Autodesk Fusion 360 part; units mm, degrees
(part 7 of 7)
  measures "d140" distance of A39.centre L1475
  measures "d141" diameter of A36
  measures "d142" distance of A36.centre L3866
  measures "d143" distance of A36.centre L1475
  measures "d144" diameter of A2
  measures "d145" distance of A0.centre L214
  measures "d146" distance of A0.centre L904
  measures "d147" diameter of A29
  measures "d148" distance of A21.centre L241
  measures "d149" distance of A21.centre L1147
  measures "d150" diameter of A17
  measures "d151" distance of A17.centre L2172
  measures "d152" distance of A17.centre L1106
  measures "d153" diameter of A69
  measures "d154" diameter of A50
  measures "d155" diameter of A63
  measures "d156" diameter of A15
  measures "d157" diameter of A47
  measures "d158" diameter of A5
  measures "d159" distance of A5.centre L1493
  measures "d160" distance of A43.centre L926
  measures "d161" distance of A15.centre L926
  measures "d162" distance of A60.centre L796
  measures "d163" distance of A68.centre L4112
  measures "d164" distance of A17.centre L1102
  measures "d165" distance of A68.centre L4388
  measures "d166" distance of A68.centre L4363
  measures "d167" distance of A49.centre L3076
  measures "d168" distance of A49.centre L3488
  measures "d169" distance of A60.centre L3636
  measures "d170" distance of A60.centre L3768
  measures "d171" distance of A15.centre L1414
  measures "d172" distance of A15.centre L1372
  measures "d173" distance of A43.centre L577
  measures "d174" distance of A43.centre L2522
  measures "d175" distance of A5.centre L729
  measures "d176" distance of A5.centre L761
  measures "d177" distance of A17.centre L1070
  measures "d178" distance of A17.centre L1079
  measures "d179" distance of A21.centre L1134
  measures "d180" distance of A21.centre L1105
  measures "d181" distance of A0.centre L205
  measures "d182" distance of A0.centre L871
  measures "d183" distance of A53.centre L2428
  measures "d184" distance of A53.centre L3199
  measures "d185" distance of A39.centre L4631
  measures "d186" distance of A39.centre L1477
  measures "d187" distance of A36.centre L1441
  measures "d188" radius of A32
  measures "d189" distance of L2406 L2562
  measures "d190" distance of L2398 L2487
  measures "d191" distance of L2399 L2562
  measures "d192" distance of L2398 L2532
  measures "d193" distance of L2406 L2546
  measures "d194" distance of L2487 L2580
  measures "d195" distance of L2490 L2532
  measures "d196" distance of L1493 L2399
sketch "Sketch3" plane through (0, 0, 0) normal (0, 0, 1) x (1, 0, 0)
  line L0 (-169.0689, -23.2426) -> (259.656, -23.2426)
  arc A0 (-174.0689, -18.2426) -> (-169.0689, -23.2426) centre (-169.0689, -18.2426) ccw
  line L1 (-174.0689, 118.4832) -> (-174.0689, -18.2426)
  arc A1 (-169.0689, 123.4832) -> (-174.0689, 118.4832) centre (-169.0689, 118.4832) ccw
  line L2 (-158.7961, 123.4832) -> (-169.0689, 123.4832)
  line L3 (259.656, 123.4832) -> (-158.7961, 123.4832)
  arc A2 (264.656, 118.4832) -> (259.656, 123.4832) centre (259.656, 118.4832) ccw
  line L4 (264.656, -18.2426) -> (264.656, 118.4832)
  arc A3 (259.656, -23.2426) -> (264.656, -18.2426) centre (259.656, -18.2426) ccw
  line L5 (260.257, 83.109) -> (260.257, -11.1417)
  line L6 (257.232, 0.4083) -> (257.232, 14.4091)
  line L7 (209.607, -9.1167) -> (195.605, -9.1167)
  line L8 (162.267, 109.6602) -> (176.267, 109.6602)
  line L9 (-166.345, 99.7592) -> (-166.345, 105.5592)
  line L10 (205.13, 81.084) -> (219.132, 81.084)
  line L11 (143.217, 95.6582) -> (157.217, 95.6582)
  line L12 (121.142, 83.109) -> (121.142, -11.1417)
  line L13 (114.998, -11.1417) -> (114.998, 83.109)
  line L14 (183.055, 83.109) -> (183.055, -11.1417)
  line L15 (179.292, -11.1417) -> (179.292, 83.109)
  line L16 (-131.2701, 111.6852) -> (-131.2701, 93.6332)
  line L17 (-149.3191, 93.6332) -> (-149.3191, 111.6852)
  line L18 (-45.545, 111.6852) -> (-45.545, 93.6332)
  line L19 (-54.069, 93.6332) -> (-54.069, 111.6852)
  line L20 (40.18, 111.6852) -> (40.18, 93.6332)
  line L21 (31.656, 93.6332) -> (31.656, 111.6852)
  line L22 (121.142, 111.6852) -> (121.142, 93.6332)
  line L23 (117.381, 93.6332) -> (117.381, 111.6852)
  line L24 (179.292, 93.6332) -> (179.292, 111.6852)
  line L25 (185.808, 109.3822) -> (198.508, 109.3822)
  line L26 (185.808, 96.3822) -> (185.808, 109.3822)
  line L27 (198.508, 96.3822) -> (185.808, 96.3822)
  line L28 (198.508, 109.3822) -> (198.508, 96.3822)
  line L29 (-152.3441, 99.7592) -> (-152.3441, 105.5592)
  line L30 (-128.2451, 105.5592) -> (-128.2451, 99.7592)
  line L31 (43.205, 99.7592) -> (43.205, 105.5592)
  line L32 (114.356, 105.5592) -> (114.356, 99.7592)
  line L33 (-57.094, 99.7592) -> (-57.094, 105.5592)
  line L34 (-42.52, 99.7592) -> (-42.52, 105.5592)
  line L35 (28.631, 105.5592) -> (28.631, 99.7592)
  line L36 (124.167, 105.5592) -> (124.167, 99.7592)
  line L37 (176.267, 105.5592) -> (176.267, 99.7592)
  line L38 (186.08, 52.1344) -> (186.08, 57.9344)
  line L39 (176.267, 57.9344) -> (176.267, 52.1344)
  line L40 (111.973, -5.0157) -> (111.973, 0.7845)
  line L41 (124.167, -5.0157) -> (124.167, 0.7845)
  line L42 (-168.37, 112.6852) -> (-150.3191, 112.6852)
  line L43 (-168.37, 92.6332) -> (-150.3191, 92.6332)
  line L44 (-130.2701, 92.6332) -> (-55.069, 92.6332)
  line L45 (-130.2701, 112.6852) -> (-55.069, 112.6852)
  line L46 (-44.545, 92.6332) -> (30.656, 92.6332)
  line L47 (-44.545, 112.6852) -> (30.656, 112.6852)
  line L48 (41.18, 92.6332) -> (116.381, 92.6332)
  line L49 (122.142, 92.6332) -> (178.292, 92.6332)
  line L50 (113.998, 84.109) -> (-168.37, 84.109)
  line L51 (41.18, 112.6852) -> (116.381, 112.6852)
  line L52 (122.142, 112.6852) -> (178.292, 112.6852)
  line L53 (259.257, 84.109) -> (184.055, 84.109)
  line L54 (178.292, 84.109) -> (122.142, 84.109)
  line L55 (259.257, -12.1417) -> (184.055, -12.1417)
  line L56 (178.292, -12.1417) -> (122.142, -12.1417)
  line L57 (113.998, -12.1417) -> (-168.37, -12.1417)
  line L58 (-169.37, -11.1417) -> (-169.37, 83.109)
  line L59 (-169.37, 93.6332) -> (-169.37, 111.6852)
  line L60 (185.808, 109.3822) -> (198.508, 96.3822)
  circle A4 centre (192.158, 102.8822) radius 3.75
  circle A5 centre (192.158, 102.8822) radius 9.25
  arc A6 (-168.37, 112.6852) -> (-169.37, 111.6852) centre (-168.37, 111.6852) ccw
  arc A7 (-169.37, 93.6332) -> (-168.37, 92.6332) centre (-168.37, 93.6332) ccw
  arc A8 (-150.3191, 92.6332) -> (-149.3191, 93.6332) centre (-150.3191, 93.6332) ccw
  arc A9 (-149.3191, 111.6852) -> (-150.3191, 112.6852) centre (-150.3191, 111.6852) ccw
  arc A10 (-130.2701, 112.6852) -> (-131.2701, 111.6852) centre (-130.2701, 111.6852) ccw
  arc A11 (-131.2701, 93.6332) -> (-130.2701, 92.6332) centre (-130.2701, 93.6332) ccw
  arc A12 (-54.069, 111.6852) -> (-55.069, 112.6852) centre (-55.069, 111.6852) ccw
  arc A13 (-55.069, 92.6332) -> (-54.069, 93.6332) centre (-55.069, 93.6332) ccw
  arc A14 (-45.545, 93.6332) -> (-44.545, 92.6332) centre (-44.545, 93.6332) ccw
  arc A15 (-44.545, 112.6852) -> (-45.545, 111.6852) centre (-44.545, 111.6852) ccw
  arc A16 (31.656, 111.6852) -> (30.656, 112.6852) centre (30.656, 111.6852) ccw
  arc A17 (30.656, 92.6332) -> (31.656, 93.6332) centre (30.656, 93.6332) ccw
  arc A18 (40.18, 93.6332) -> (41.18, 92.6332) centre (41.18, 93.6332) ccw
  arc A19 (41.18, 112.6852) -> (40.18, 111.6852) centre (41.18, 111.6852) ccw
  arc A20 (117.381, 111.6852) -> (116.381, 112.6852) centre (116.381, 111.6852) ccw
  arc A21 (116.381, 92.6332) -> (117.381, 93.6332) centre (116.381, 93.6332) ccw
  arc A22 (121.142, 93.6332) -> (122.142, 92.6332) centre (122.142, 93.6332) ccw
  arc A23 (122.142, 112.6852) -> (121.142, 111.6852) centre (122.142, 111.6852) ccw
  arc A24 (179.292, 111.6852) -> (178.292, 112.6852) centre (178.292, 111.6852) ccw
  arc A25 (178.292, 92.6332) -> (179.292, 93.6332) centre (178.292, 93.6332) ccw
  arc A26 (184.055, 84.109) -> (183.055, 83.109) centre (184.055, 83.109) ccw
  arc A27 (260.257, 83.109) -> (259.257, 84.109) centre (259.257, 83.109) ccw
  arc A28 (259.257, -12.1417) -> (260.257, -11.1417) centre (259.257, -11.1417) ccw
  arc A29 (183.055, -11.1417) -> (184.055, -12.1417) centre (184.055, -11.1417) ccw
  arc A30 (179.292, 83.109) -> (178.292, 84.109) centre (178.292, 83.109) ccw
  arc A31 (178.292, -12.1417) -> (179.292, -11.1417) centre (178.292, -11.1417) ccw
  arc A32 (121.142, -11.1417) -> (122.142, -12.1417) centre (122.142, -11.1417) ccw
  arc A33 (122.142, 84.109) -> (121.142, 83.109) centre (122.142, 83.109) ccw
  arc A34 (114.998, 83.109) -> (113.998, 84.109) centre (113.998, 83.109) ccw
  arc A35 (113.998, -12.1417) -> (114.998, -11.1417) centre (113.998, -11.1417) ccw
  arc A36 (-169.37, -11.1417) -> (-168.37, -12.1417) centre (-168.37, -11.1417) ccw
  arc A37 (-168.37, 84.109) -> (-169.37, 83.109) centre (-168.37, 83.109) ccw
  line L61 (-152.3441, 109.6602) -> (-166.345, 109.6602)
  line L62 (-166.345, 95.6582) -> (-152.3441, 95.6582)
  line L63 (-171.5689, 114.6832) -> (262.156, 114.6832)
  line L64 (-171.5689, 114.6832) -> (-171.5689, -14.4426)
  line L65 (262.156, -14.4426) -> (-171.5689, -14.4426)
  line L66 (262.156, 114.6832) -> (262.156, -14.4426)
  dimension "d197" = 3.025
  dimension "d198" = 3.025
  dimension "d199" = 3.025
  dimension "d200" = 3.025
  dimension "d201" = 3.025
  dimension "d202" = 3.025
  dimension "d203" = 3.025
  dimension "d204" = 3.025
  dimension "d205" = 3.025
  dimension "d206" = 3.025
  dimension "d207" = 3.025
  dimension "d208" = 3.025
  dimension "d209" = 3.025
  dimension "d210" = 3.025
  dimension "d211" = 3.025
  dimension "d212" = 3.025
  dimension "d213" = 3.025
  dimension "d214" = 3.025
  dimension "d215" = 3.025
  dimension "d216" = 7.5
  dimension "d218" = 18.5
  dimension "d219" = 1
  constraint horizontal L42
  constraint vertical L5
  constraint horizontal L55
  constraint vertical L58
  constraint horizontal L43
  constraint horizontal L53
  constraint vertical L12
  constraint vertical L13
  constraint vertical L14
  constraint vertical L15
  constraint vertical L16
  constraint vertical L17
  constraint vertical L18
  constraint vertical L19
  constraint vertical L20
  constraint vertical L21
  constraint vertical L22
  constraint vertical L23
  constraint vertical L24
  constraint collinear L42 L45
  constraint collinear L43 L44
  constraint collinear L44 L46
  constraint collinear L45 L47
  constraint collinear L46 L48
  constraint collinear L47 L51
  constraint collinear L48 L49
  constraint collinear L50 L54
  constraint collinear L51 L52
  constraint collinear L53 L54
  constraint collinear L55 L56
  constraint collinear L56 L57
  constraint collinear L58 L59
  constraint coincident L25.start L26.end
  constraint coincident L27.start L28.end
  constraint midpoint L60 A4.centre
  constraint tangent L42 A6
  constraint tangent L59 A6
  constraint tangent L43 A7
  constraint tangent L59 A7
  constraint equal A6 A7
  constraint tangent L17 A8
  constraint tangent L43 A8
  constraint equal A6 A8
  constraint tangent L17 A9
  constraint tangent L42 A9
  constraint equal A6 A9
  constraint tangent L16 A10
  constraint tangent L45 A10
  constraint equal A6 A10
  constraint tangent L16 A11
  constraint tangent L44 A11
  constraint equal A6 A11
  constraint tangent L19 A12
  constraint tangent L45 A12
  constraint equal A6 A12
  constraint tangent L19 A13
  constraint tangent L44 A13
  constraint equal A6 A13
  constraint tangent L18 A14
  constraint tangent L46 A14
  constraint equal A6 A14
  constraint tangent L18 A15
  constraint tangent L47 A15
  constraint equal A6 A15
  constraint tangent L21 A16
  constraint tangent L47 A16
  constraint equal A6 A16
  constraint tangent L21 A17
  constraint tangent L46 A17
  constraint equal A6 A17
  constraint tangent L20 A18
  constraint tangent L48 A18
  constraint equal A6 A18
  constraint tangent L20 A19
  constraint tangent L51 A19
  constraint equal A6 A19
  constraint tangent L23 A20
  constraint tangent L51 A20
  constraint equal A6 A20
  constraint tangent L23 A21
  constraint tangent L48 A21
  constraint equal A6 A21
  constraint tangent L22 A22
  constraint tangent L49 A22
  constraint equal A6 A22
  constraint tangent L22 A23
  constraint tangent L52 A23
  constraint equal A6 A23
  constraint tangent L52 A24
  constraint tangent L24 A24
  constraint equal A6 A24
  constraint tangent L49 A25
  constraint tangent L24 A25
  constraint equal A6 A25
  constraint tangent L53 A26
  constraint tangent L14 A26
  constraint equal A6 A26
  constraint tangent L53 A27
  constraint tangent L5 A27
  constraint equal A6 A27
  constraint tangent L5 A28
  constraint tangent L55 A28
  constraint equal A6 A28
  constraint tangent L55 A29
  constraint tangent L14 A29
  constraint equal A6 A29
  constraint tangent L15 A30
  constraint tangent L54 A30
  constraint equal A6 A30
  constraint tangent L15 A31
  constraint tangent L56 A31
  constraint equal A6 A31
  constraint tangent L56 A32
  constraint tangent L12 A32
  constraint equal A6 A32
  constraint tangent L12 A33
  constraint tangent L54 A33
  constraint equal A6 A33
  constraint tangent L50 A34
  constraint tangent L13 A34
  constraint equal A6 A34
  constraint tangent L57 A35
  constraint tangent L13 A35
  constraint equal A6 A35
  constraint tangent L57 A36
  constraint tangent L58 A36
  constraint equal A6 A36
  constraint tangent L58 A37
  constraint tangent L50 A37
  constraint equal A6 A37
  measures "d197" distance of L5 L6
  measures "d198" distance of L7 L55
  measures "d199" distance of L8 L52
  measures "d200" distance of L9 L59
  measures "d201" distance of L10 L53
  measures "d202" distance of L11 L49
  measures "d203" distance of L17 L29
  measures "d204" distance of L16 L30
  measures "d205" distance of L20 L31
  measures "d206" distance of L23 L32
  measures "d207" distance of L19 L33
  measures "d208" distance of L18 L34
  measures "d209" distance of L21 L35
  measures "d210" distance of L22 L36
  measures "d211" distance of L24 L37
  measures "d212" distance of L14 L38
  measures "d213" distance of L15 L39
  measures "d214" distance of L13 L40
  measures "d215" distance of L12 L41
  measures "d216" diameter of A4
  measures "d218" diameter of A5
  measures "d219" radius of A6
extrude "Extrude2" add sketch "Sketch1" along normal blind 4.5 contours A12 A13 L19 L32 L42 L48 A44 A52 L78 L89 makes body 1
extrude "Extrude3" add sketch "Sketch1" along normal blind 3 from surface at 4.5 separate body contours L0 L2 L4 A5 A7 A28 A35 L90 A97 L124 L125 | A1 L5 A10 L16 A19 A22 L65 L90 L122 A96 L123 | L90 A97 L124 L125 | L90 L122 A96 L123 | L49 A42 A43 L54 A55 L67 A57 L90 L120 A95 L121 | L90 L120 A95 L121 | A4 A11 L10 L12 A14 A18 L33 L95 L102 L103 A86 | L95 L102 L103 A86 | L72 L73 A62 A64 A67 L84 A71 L90 L118 A94 L119 | L90 L118 A94 L119 | A21 A24 L25 L26 A34 A36 L36 L95 L104 A87 L105 | L95 L104 A87 L105 | L37 A41 A46 L59 A51 L63 A59 L90 A93 L116 L117 | L90 A93 L116 L117 | L22 L27 A27 A29 L29 A31 A32 L95 L106 A88 L107 | L95 L106 A88 L107 | L41 L43 A40 A49 A50 L64 A58 L90 L114 A92 L115 | L90 L114 A92 L115 | L74 L75 A63 L77 A65 A68 A69 L95 L108 A89 L109 | L95 L108 A89 L109 | A75 L93 L95 A81 A82 L99 L100 A85 L110 A90 L111 | L57 A73 L87 L88 A76 A77 L95 A80 L112 A91 L113 | L95 L110 A90 L111 | L95 L112 A91 L113 | A0 | A2 | A3 | A6 | A8 | A9 | A12 A13 L19 L32 L42 L48 A44 A52 L78 L89 | A15 | A16 | A17 | A20 | A23 | A25 | A26 | A30 | A33 | A37 | A38 | A39 | A45 | A47 | A48 | A53 | A54 | A56 | A60 | A61 | A66 | A70 | A72 | A74 | A78 | A79 | A83 | A84 | A98 | A99 makes body 2
extrude "Extrude4" add sketch "Sketch3" along normal blind 6 from surface at 1.5 separate body contours L63 L64 L65 L66 makes body 3
combine "Combine1" operation add target body 3 tool bodies 2 1
extrude "Extrude5" add sketch "Sketch3" along normal blind 3 from surface at 1.5 contours L26 L27 L60 A4 | L25 L28 L60 A4 | A5 bodies 3
